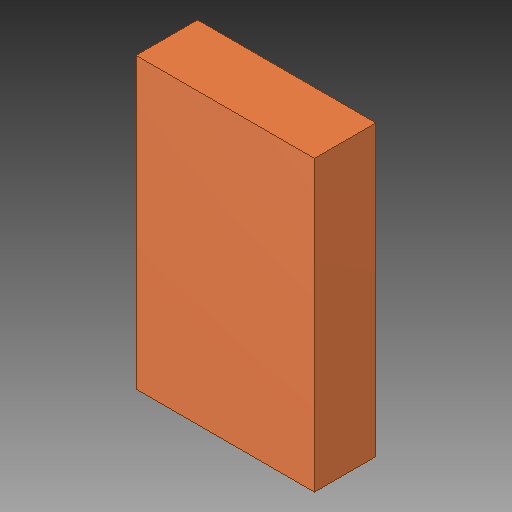
# Autodesk Inventor part: LED_IC_1_STATUS_P-LCC-2
Saved by Autodesk Inventor 2017 (Build 210142000, 142)
## iProperties
Created: 2019-06-13
Part Number: LED_IC_1_STATUS_P-LCC-2
Material: Generic
Document SubType Name: Modeling
Designer: Marc
Density: 1 g/cm^3
Appearance: P-LCC-2, LED_IC_1_STATUS_P-LCC-2
Author: Marc
Autodesk Inventor part; units mm, degrees
ref_plane "YZ Plane" through (0, 0, 0) normal (1, 0, 0) x (0, 1, 0)
ref_plane "XZ Plane" through (0, 0, 0) normal (0, 1, 0) x (-1, 0, 0)
ref_plane "XY Plane" through (0, 0, 0) normal (0, 0, 1) x (1, 0, 0)
sketch "P-LCC-2, LED_IC_1_STATUS_P-LCC-2_42" plane through (0, 0, 0) normal (0, 0, 1) x (1, 0, 0)
  line L0 (-1.5016, 2.35) -> (1.4, 2.35)
  line L1 (1.4, 2.35) -> (1.4, -2.35)
  line L2 (1.4, -2.35) -> (-1.5016, -2.35)
  line L3 (-1.5016, -2.35) -> (-1.5016, 2.35)
  constraints: 8 end point
extrude "Extrusion1" add sketch "P-LCC-2, LED_IC_1_STATUS_P-LCC-2_42" along normal blind 1
body "Solid1"
